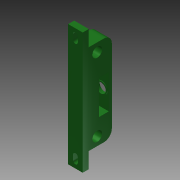
# Autodesk Inventor part: Part8
Saved by Autodesk Inventor 2015 (Build 190159000, 159)
## iProperties
Created: 2015-07-07
Part Number: Part8
Material: ABS Plastic
Document SubType Name: Modeling
Designer: hp
Density: 1.06 g/cm^3
Appearance: Smooth - Dark Forest Green
Author: hp
Autodesk Inventor part; units mm, degrees
ref_plane "YZ Plane" through (0, 0, 0) normal (1, 0, 0) x (0, 1, 0)
ref_plane "XZ Plane" through (0, 0, 0) normal (0, 1, 0) x (-1, 0, 0)
ref_plane "XY Plane" through (0, 0, 0) normal (0, 0, 1) x (1, 0, 0)
sketch "Sketch1" plane through (0, 0, 0) normal (1, 0, 0) x (0, 1, 0)
  line L0 (0, 50) -> (0, -50)
  line L1 (0, -50) -> (5, -50)
  line L2 (5, -50) -> (5, -37)
  line L3 (5, -37) -> (17.41, -37)
  line L4 (24, -30.41) -> (24, 30.41)
  line L5 (17.41, 37) -> (5, 37)
  line L6 (5, 37) -> (5, 50)
  line L7 (5, 50) -> (0, 50)
  line L8 (21.5, 11) -> (13.5, 11)
  line L9 (13.5, 11) -> (13.5, -17)
  line L10 (13.5, -17) -> (21.5, -17)
  line L11 (21.5, -17) -> (21.5, 11)
  circle A0 centre (11.9411, 30) radius 4
  circle A1 centre (11.9411, -30) radius 4
  arc A2 (24, 30.41) -> (17.41, 37) centre (17.41, 30.41) ccw
  arc A3 (17.41, -37) -> (24, -30.41) centre (17.41, -30.41) ccw
  point P0 (0, 0)
  point P1 (24, -37)
  point P2 (0, 0)
  dimension "d0" = 100
  dimension "d1" = 5
  dimension "d2" = 13
  dimension "d3" = 13
  dimension "d4" = 19
  dimension "d5" = 28
  dimension "d6" = 26
  dimension "d7" = 8
  dimension "d8" = 2.5
  dimension "d9" = 8
  dimension "d10" = 60
  dimension "d11" = 30
  dimension "d12" = 6.59
  constraints: 24 end point, 7 perpendicular, 4 centre point, 4 point on circle, 4 point on line, 4 tangent, 2 equal radius, 2 parallel, 2 vertical alignment, 1 coincident, 1 horizontal, 1 midpoint, 1 vertical
  measures "d0" distance of L0.start L0.end
  measures "d1" distance of L0.end L1.end
  measures "d2" distance of L1.end L2.end
  measures "d3" distance of L5.end L6.end
  measures "d4" distance of L2.end point (24, -37)
  measures "d5" distance of L10.end L8.start
  measures "d6" distance between parallel lines of L5 L8
  measures "d7" distance of L9.end L10.end
  measures "d8" distance between parallel lines of L4 L11
  measures "d9" diameter of A0
  measures "d10" distance of A1.centre A0.centre
  measures "d11" vertical distance of point (0, 0) A0.centre
  measures "d12" radius of A2
extrude "Extrusion1" add sketch "Sketch1" along normal blind 12
sketch "Sketch2" plane through (0, 24, 30.41) normal (0, 1, 0) x (1, 0, 0)
  circle A0 centre (6, 33.41) radius 4
  line L0 (0, -6.59) -> (12, -6.59) projected
  point P0 (0, 30.41)
  point P1 (6, -6.59)
  dimension "d15" = 40
  dimension "d16" = 8
  constraints: 1 centre point, 1 midpoint, 1 vertical alignment
  measures "d15" distance from line of L0 A0.centre
  measures "d16" diameter of A0
extrude "Extrusion2" cut sketch "Sketch2" against normal blind 20
sketch "Sketch3" plane through (0, 0, -50) normal (0, -1, 0) x (1, 0, 0)
  line L0 (4, 95) -> (4, 91)
  line L1 (8, 91) -> (8, 95)
  arc A0 (4, 91) -> (8, 91) centre (6, 91) ccw
  arc A1 (8, 95) -> (4, 95) centre (6, 95) ccw
  line L2 (0, 100) -> (12, 100) projected
  line L3 (0, 100) -> (0, 0) projected
  line L4 (4, 9) -> (4, 5)
  line L5 (8, 5) -> (8, 9)
  arc A2 (4, 5) -> (8, 5) centre (6, 5) ccw
  arc A3 (8, 9) -> (4, 9) centre (6, 9) ccw
  line L6 (0, 0) -> (12, 0) projected
  point P0 (0, 50)
  dimension "d19" = 4
  dimension "d20" = 4
  dimension "d21" = 5
  dimension "d22" = 6
  dimension "d23" = 4
  dimension "d24" = 4
  dimension "d25" = 5
  constraints: 8 end point, 8 point on circle, 8 tangent, 4 centre point, 2 parallel, 2 vertical, 1 vertical alignment
  measures "d19" distance of L1.start L0.end
  measures "d20" distance of L0.end L0.start
  measures "d21" distance from line of L2 A1.centre
  measures "d22" distance from line of L3 A1.centre
  measures "d23" distance of L5.start L4.end
  measures "d24" distance of L4.end L4.start
  measures "d25" distance from line of L6 A2.centre
extrude "Extrusion3" cut sketch "Sketch3" against normal up to next
sketch "Sketch5" plane through (0, 13.5, 11) normal (0, 1, 0) x (1, 0, 0)
  circle A0 centre (6, 14) radius 4 projected
  circle A1 centre (6, 14) radius 5
  point P0 (0, 11)
  dimension "d28" = 10
  constraints: 1 centre point, 1 coincident
  measures "d28" diameter of A1
extrude "Extrusion4" add sketch "Sketch5" along normal blind 0.5
pattern_linear "Rectangular Pattern1" count 2 spacing 7.5 along (0, 1, 0) of "Extrusion4"
equation "\"d3\" = d2"
body "Solid1"
